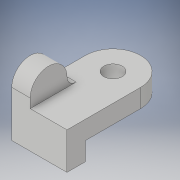
# Autodesk Inventor part: Part7
Saved by Autodesk Inventor 2017 (Build 210142000, 142)
## iProperties
Created: 2016-11-03
Part Number: Part7
Material: Generic
Document SubType Name: Modeling
Designer: s411888
Density: 1 g/cm^3
Appearance: Default
Author: s411888
Autodesk Inventor part; units mm, degrees
ref_plane "YZ Plane" through (0, 0, 0) normal (1, 0, 0) x (0, 1, 0)
ref_plane "XZ Plane" through (0, 0, 0) normal (0, 1, 0) x (-1, 0, 0)
ref_plane "XY Plane" through (0, 0, 0) normal (0, 0, 1) x (1, 0, 0)
sketch "Sketch1" plane through (0, 0, 0) normal (1, 0, 0) x (0, 1, 0)
  line L0 (-0.02, 31.5145) -> (-25.42, 31.5145)
  line L1 (-25.42, 31.5145) -> (-25.42, 18.8145)
  line L2 (-25.42, 18.8145) -> (-0.02, 18.8145)
  line L3 (-0.02, 18.8145) -> (-0.02, 31.5145)
  line L4 (-0.02, 31.5145) -> (-12.72, 31.5145)
  line L5 (-12.72, 31.5145) -> (-12.72, -19.2855)
  line L6 (-12.72, -19.2855) -> (-0.02, -19.2855)
  line L7 (-0.02, -19.2855) -> (-0.02, 31.5145)
  point P0 (0, 0)
  dimension "d0" = 25.4
  dimension "d1" = 12.7
  dimension "d2" = 12.7
  dimension "d3" = 50.8
  constraints: 16 end point, 4 parallel, 2 horizontal, 2 perpendicular
  measures "d0" distance of L2.end L1.end
  measures "d1" distance of L1.end L0.end
  measures "d2" distance of L6.end L5.end
  measures "d3" distance of L5.end L4.end
extrude "Extrusion1" add sketch "Sketch1" along normal blind 38.1
sketch "Sketch2" plane through (0, -0.02, 31.5145) normal (0, 1, 0) x (1, 0, 0)
  line L0 (0, 50.8) -> (38.1, 50.8) projected
  line L1 (38.1, 50.8) -> (19.05, 50.8)
  circle A0 centre (19.05, 50.8) radius 19.05
  line L2 (0, 50.8) -> (0, 0) projected
  line L3 (0, 50.8) -> (38.1, 50.8)
  line L4 (0, 50.8) -> (38.1, 50.8)
  point P0 (0, 31.5145)
  dimension "d7" = 38.1
  constraints: 6 end point, 2 horizontal, 1 centre point, 1 coincident, 1 collinear
  measures "d7" diameter of A0
extrude "Extrusion2" add sketch "Sketch2" against normal blind 12.7
sketch "Sketch3" plane through (0, -0.02, 31.5145) normal (0, 1, 0) x (1, 0, 0)
  line L0 (38.1, 12.7) -> (38.1, 50.8) projected
  line L1 (38.1, 50.8) -> (19.05, 50.8)
  circle A0 centre (19.05, 50.8) radius 6.35
  point P0 (0, 31.5145)
  dimension "d10" = 19.05
  dimension "d11" = 12.7
  constraints: 2 end point, 1 centre point, 1 coincident, 1 horizontal
  measures "d10" distance of L0.end L1.end
  measures "d11" diameter of A0
extrude "Extrusion3" cut sketch "Sketch3" against normal blind 12.7
sketch "Sketch4" plane through (0, -0.02, 31.5145) normal (0, 1, 0) x (1, 0, 0)
  line L0 (0, 0) -> (38.1, 0) projected
  line L1 (0, 0) -> (12.7, 0)
  line L2 (12.7, 0) -> (12.7, 25.4)
  line L3 (12.7, 25.4) -> (0, 25.4)
  line L4 (0, 25.4) -> (0, 0)
  point P0 (0, 31.5145)
  dimension "d14" = 12.7
  dimension "d15" = 25.4
  constraints: 8 end point, 2 parallel, 1 horizontal, 1 perpendicular
  measures "d14" distance of L3.end L2.end
  measures "d15" distance of L2.end L1.end
extrude "Extrusion4" add sketch "Sketch4" along normal blind 6.35
sketch "Sketch5" plane through (12.7, -0.02, 31.5145) normal (1, 0, 0) x (0, 0, -1)
  line L0 (0, 0) -> (0, 6.35) projected
  line L1 (0, 6.35) -> (25.4, 6.35) projected
  circle A0 centre (12.7, 6.35) radius 12.7
  point P0 (31.5145, 0.02)
  dimension "d19" = 25.4
  constraints: 1 centre point
  measures "d19" diameter of A0
extrude "Extrusion5" add sketch "Sketch5" against normal blind 12.7
fillet "Fillet1" radius 6.35 1 edges at (6.35, -0.02, 6.1145)
body "Solid1"
